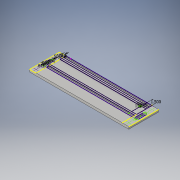
# Autodesk Inventor part: Fixture Base
Saved by Autodesk Inventor 2016 (Build 200138000, 138)
## iProperties
Created: 2016-04-07
Part Number: Fixture Base
Material: Generic
Document SubType Name: Modeling
Designer: Sam Clay
Density: 1 g/cm^3
Appearance: Default
Author: Sam Clay
Autodesk Inventor part; units mm, degrees
ref_plane "YZ Plane" through (0, 0, 0) normal (1, 0, 0) x (0, 1, 0)
ref_plane "XZ Plane" through (0, 0, 0) normal (0, 1, 0) x (-1, 0, 0)
ref_plane "XY Plane" through (0, 0, 0) normal (0, 0, 1) x (1, 0, 0)
sketch "Base Sketch" plane through (0, 0, 0) normal (0, 1, 0) x (-1, 0, 0)
  line L0 (0, 0) -> (660.4, 0)
  line L1 (660.4, 0) -> (660.4, 228.6)
  line L2 (660.4, 228.6) -> (0, 228.6)
  line L3 (0, 228.6) -> (0, 0)
  line L4 (0, 228.6) -> (-50.8, 228.6)
  line L5 (-50.8, 228.6) -> (-50.8, 0)
  line L6 (-50.8, 0) -> (0, 0)
  line L7 (0, 0) -> (0, 228.6)
  line L8 (660.4, 228.6) -> (711.2, 228.6)
  line L9 (711.2, 228.6) -> (711.2, 0)
  line L10 (711.2, 0) -> (660.4, 0)
  line L11 (660.4, 0) -> (660.4, 228.6)
  dimension "d0" = 660.4
  dimension "d1" = 228.6
  dimension "d87" = 50.8
  dimension "d88" = 50.8
  constraints: 24 end point, 6 parallel, 3 horizontal, 3 perpendicular, 1 point on line
  measures "d0" distance of L2.end L1.end
  measures "d1" distance of L1.end L0.end
  measures "d87" distance of L6.end L5.end
  measures "d88" distance of L9.end L10.end
extrude "Base" add sketch "Base Sketch" along normal blind 19.05 contours L3 L2 L1 L0
sketch "Tracks Sketch" plane through (0, 19.05, 0) normal (0, 1, 0) x (1, 0, 0)
  line L0 (0, 0) -> (-660.4, 0) projected
  line L1 (-660.4, 0) -> (-660.4, -228.6) projected
  line L2 (0, 0) -> (-660.4, 0)
  line L3 (-660.4, 0) -> (-660.4, -20.066)
  line L4 (-660.4, -20.066) -> (0, -20.066)
  line L5 (0, -20.066) -> (0, 0)
  line L6 (0, 0) -> (-38.1, 0)
  line L7 (-38.1, 0) -> (-38.1, -118.491)
  line L8 (-38.1, -118.491) -> (0, -118.491)
  line L9 (0, -118.491) -> (0, 0)
  line L10 (-38.1, -151.003) -> (-660.4, -151.003)
  line L11 (-660.4, -151.003) -> (-660.4, -131.191)
  line L12 (-660.4, -131.191) -> (-38.1, -131.191)
  line L13 (-38.1, -131.191) -> (-38.1, -151.003)
  line L14 (0, -45.466) -> (-660.4, -45.466)
  line L15 (-660.4, -45.466) -> (-660.4, -32.766)
  line L16 (-660.4, -32.766) -> (0, -32.766)
  line L17 (0, -32.766) -> (0, -45.466)
  line L18 (-38.1, -40.5821) -> (-33.2161, -45.466)
  line L19 (-38.1, -40.5821) -> (-45.0069, -40.5821) construction
  circle A0 centre (-41.4506, -48.8166) radius 8.89
  line L20 (-660.4, -0.254) -> (0, -0.254)
  line L21 (0, -228.6) -> (0, 0) projected
  line L22 (-38.1, -118.491) -> (-660.4, -118.491)
  line L23 (-660.4, -151.7967) -> (0, -151.7968)
  line L24 (-38.1, -151.003) -> (0, -151.003)
  line L25 (-38.1, -131.191) -> (0, -131.191)
  point P0 (-38.1, -20.066)
  point P1 (-38.1, -45.466)
  point P2 (-38.1, -45.466)
  point P3 (-38.1, -0.254)
  dimension "d5" = 38.1
  dimension "d75" = 19.812
  dimension "d76" = 12.7
  dimension "d77" = 12.7
  dimension "d78" = 12.7
  dimension "d79" = 73.025
  dimension "d83" = 135
  dimension "d84" = 17.78
  dimension "d101" = 0.254
  dimension "d102" = 19.812
  dimension "d109" = 0.7937
  constraints: 46 end point, 20 point on line, 8 parallel, 8 perpendicular, 6 horizontal, 4 coincident, 2 point on circle, 1 centre point, 1 equal length
  measures "d5" distance of L8.end L7.end
  measures "d75" distance of L10.end L11.end
  measures "d76" distance from line of L8.end L12
  measures "d77" distance of L14.end L15.end
  measures "d78" distance between parallel lines of L4 L16
  measures "d79" distance from line of L14 L7.end
  measures "d83" angle of L19 L18
  measures "d84" diameter of A0
  measures "d101" distance between parallel lines of L0 L20
  measures "d102" distance between parallel lines of L4 L20
  measures "d109" distance between parallel lines of L23 L10
extrude "Track Separator" cut sketch "Tracks Sketch" against normal blind 0.0254 contours L21 L23 L1 L10 L24
extrude "Pocket side" cut sketch "Tracks Sketch" against normal blind 3.175 contours L18 L14 L7 | A0 L18 | L7 L14 A0 | A0 L7 L14 | L14 A0 L7 L22 L1 | L7 A0 L14
extrude "Tracks" cut sketch "Tracks Sketch" against normal blind 9.8425 contours L5 L4 L7 L20 | L7 L4 L1 L20 | L21 L24 L13 L25 | L13 L10 L1 L12
extrude "Lower Level" add sketch "Base Sketch" along normal blind 17.78 contours L6 L5 L4 L3 | L1 L8 L9 L10
sketch "Handle Sketch" plane through (0, 17.78, 0) normal (0, 1, 0) x (1, 0, 0)
  line L0 (-660.4, 0) -> (-711.2, 0) projected
  line L1 (-711.2, 0) -> (-711.2, -228.6) projected
  line L2 (50.8, -228.6) -> (50.8, 0) projected
  line L3 (-711.2, -228.6) -> (-660.4, -228.6) projected
  line L4 (25.4, -83.6181) -> (25.4, -142.6126) construction
  line L5 (12.7, -83.6181) -> (12.7, -142.6126)
  line L6 (38.1, -142.6126) -> (38.1, -83.6181)
  arc A0 (38.1, -83.6181) -> (12.7, -83.6181) centre (25.4, -83.6181) ccw
  arc A1 (12.7, -142.6126) -> (38.1, -142.6126) centre (25.4, -142.6126) ccw
  line L7 (-685.8, -83.6181) -> (-685.8, -142.6126) construction
  line L8 (-698.5, -83.6181) -> (-698.5, -142.6126)
  line L9 (-673.1, -142.6126) -> (-673.1, -83.6181)
  arc A2 (-673.1, -83.6181) -> (-698.5, -83.6181) centre (-685.8, -83.6181) ccw
  arc A3 (-698.5, -142.6126) -> (-673.1, -142.6126) centre (-685.8, -142.6126) ccw
  point P0 (0, 0)
  point P1 (-685.8, -25.4)
  point P2 (-685.8, -63.5)
  point P3 (-685.8, -165.1)
  point P4 (-622.3, 0)
  point P5 (25.4, -203.2)
  point P6 (25.4, -165.1)
  point P7 (25.4, -25.4)
  point P8 (-685.8, -203.2)
  point P9 (25.4, -63.5)
  point P10 (25.4, -113.1154)
  point P11 (-685.8, -113.1154)
  dimension "d91" = 25.4
  dimension "d97" = 38.1
  dimension "d99" = 38.1
  dimension "d100" = 25.4
  dimension "d103" = 25.4
  dimension "d104" = 25.4
  dimension "d105" = 25.4
  dimension "d106" = 25.4
  dimension "d107" = 25.4
  dimension "d108" = 25.4
  dimension "d114" = 12.7
  dimension "d115" = 25.4
  dimension "d116" = 25.4
  dimension "d117" = 25.4
  constraints: 16 end point, 8 point on circle, 8 tangent, 4 centre point, 2 midpoint, 2 parallel, 2 vertical, 2 vertical alignment
  measures "d91" distance from line of point (-685.8, -25.4) L0
  measures "d97" distance of point (-685.8, -63.5) point (-685.8, -25.4)
  measures "d99" distance of point (-685.8, -165.1) point (-685.8, -203.2)
  measures "d100" distance from line of L3 point (-685.8, -203.2)
  measures "d103" distance from line of point (-685.8, -63.5) L1
  measures "d104" distance from line of L1 point (-685.8, -25.4)
  measures "d105" distance from line of L1 point (-685.8, -165.1)
  measures "d106" distance from line of L1 point (-685.8, -203.2)
  measures "d107" distance from line of L2 point (25.4, -25.4)
  measures "d108" distance from line of L2 point (25.4, -63.5)
  measures "d114" distance between parallel lines of L6 L4
  measures "d115" diameter of A3
  measures "d116" distance from line of L1 L7.start
  measures "d117" distance from line of L2 L4.start
sketch "Origin Sketch" plane through (0, 19.05, 0) normal (0, 1, 0) x (1, 0, 0)
  point P0 (0, 0)
  point P1 (-38.1, -45.466)
  point P2 (-38.1, -45.466)
  constraints: 1 coincident
extrude "Handles" cut sketch "Handle Sketch" against normal through all
equation "\"d104\" = d103"
equation "\"d105\" = d103"
equation "\"d106\" = d103"
equation "\"d107\" = d103"
equation "\"d108\" = d103"
body "Solid1"
